spitzbubenschneider (Autodesk Fusion 360 design; units mm, degrees)
Autodesk Fusion 360 part; units mm, degrees
sketch "Sketch1" plane through (0, 0, 0) normal (0, 1, 0) x (1, 0, 0)
  circle A0 centre (0, 0) radius 27.5
  circle A1 centre (0, 0) radius 26.7
  circle A2 centre (14, 0) radius 4.05
  circle A3 centre (14, 0) radius 3.25
  line L0 (0, 0) -> (26.7, 0)
  line L1 (0, 0) -> (14, 0)
  circle A4 centre (14, 0) radius 6.45
  dimension "d1" = 55
  dimension "d2" = 0.8
  dimension "d3" = 0.8
  dimension "d4" = 14
  dimension "d5" = 6.5
  dimension "d43" = 2.4
  constraint coincident A0.centre A1.centre
  constraint concentric A2 A3
  constraint coincident A1 L0.end
  constraint horizontal L0
  constraint coincident A2.centre A3.centre
  constraint collinear L0 L1
  constraint concentric A3 A4
  measures "d1" diameter of A0
  measures "d2" distance of A0 A1
  measures "d3" distance of A2 A3
  measures "d4" distance of A0.centre A2.centre
  measures "d5" diameter of A3
  measures "d43" distance of A2 A4
extrude "Extrude1" add sketch "Sketch1" along normal blind 15 contours A0 | A2 A3 L0 L1 | A2 A3 L0 L1 makes body 1 at (27.3633, 10, 2.7381) makes body 2 at (18.0299, 5, 0.4032)
sketch "Sketch2" plane through (0, 0, 0) normal (0, 0, 1) x (1, 0, 0)
  line L0 (0, 0) -> (27.3, 0)
  line L1 (17.45, 0) -> (17.45, 3.4)
  line L2 (17.45, 3.4) -> (27.3, 0)
  line L3 (27.3, 0) -> (27.3, 3.4)
  line L4 (27.3, 3.4) -> (17.45, 3.4)
  line L5 (0, 0) -> (0, 3.4)
  line L6 (0, 3.4) -> (10.5, 3.4)
  line L7 (10.5, 3.4) -> (10.5, 0)
  dimension "d10" = 3.4
  dimension "d11" = 27.3
  dimension "d12" = 17.45
  dimension "d13" = 10.5
  constraint coincident L0.start L5.start
  constraint horizontal L0
  constraint coincident L0 L1.start
  constraint perpendicular L0 L1
  constraint perpendicular L0 L3
  constraint parallel L0 L4
  constraint perpendicular L0 L5
  constraint perpendicular L5 L6
  constraint coincident L0 L7.end
  constraint perpendicular L0 L7
  constraint collinear L4 L6
  measures "d10" distance of L1.start L1.end
  measures "d11" distance of L0.start L0.end
  measures "d12" distance of L0.start L1
  measures "d13" distance of L0.start L7
extrude "Extrude2" add sketch "Sketch2" along normal mid plane 2 separate body contours L0 L1 L2 | L2 L3 L4 makes body 3
pattern_circular "C-Pattern2" count 3 over 360 about axis through (0, 1.75, 0) along (0, 1, 0) of "Extrude1", "Extrude2" makes body 4 at (-11.3104, 5, -25.0664) makes body 5 at (-9.3642, 10, -15.4127) makes body 6 at (-9.5006, 1.1333, -18.4556) makes body 7 at (-16.053, 10, 22.3283) makes body 8 at (-8.6657, 10, 15.816) makes body 9 at (-11.2327, 1.1333, 17.4556)
sketch "Sketch4" plane through (0, 0, 0) normal (0, 0, 1) x (1, 0, 0)
  line L0 (0, 3.4) -> (-27.3, 3.4)
  line L1 (-27.3, 3.4) -> (-27.3, 0)
  line L2 (-27.3, 0) -> (0, 0)
  line L3 (0, 3.4) -> (0, 0)
  line L4 (-15, 0) -> (-15, 3.4)
  dimension "d20" = 3.4
  dimension "d22" = 27.3
  dimension "d42" = 15
  constraint vertical L1
  constraint coincident L2.end L3.end
  constraint perpendicular L1 L2
  constraint perpendicular L2 L3
  constraint coincident L2 L4.start
  constraint coincident L0 L4.end
  constraint perpendicular L0 L4
  measures "d20" distance of L0.end L1.end
  measures "d22" distance of L1 L3
  measures "d42" distance of L3 L4
extrude "Extrude3" add sketch "Sketch4" along normal mid plane 1.6 separate body contours L0 L1 L2 L4 makes body 10
pattern_circular "C-Pattern3" count 3 over 360 about axis through (0, 1.75, 0) along (0, 1, 0) of "Extrude3" makes body 11 at (10.2428, 2.2667, 16.1411) makes body 12 at (8.8572, 2.2667, -16.9411)
combine "Combine1" operation add target body 1 tool bodies 11 12 3 4 5 6 7 8 9 10 2
sketch "Sketch5" plane through (0, 0, 0) normal (0, 1, 0) x (1, 0, 0)
  circle A0 centre (0, 0) radius 27.375 construction
  circle A1 centre (0, 0) radius 27.375
  constraint coincident A0.centre A1.centre
sketch "Sketch6" plane through (0, 0, 0) normal (0, -1, 0) x (1, 0, 0)
  line L0 (8.1928, 12.5904) -> (14.0368, 22.7125)
  arc A0 (26.6813, 1) -> (14.0368, 22.7125) centre (0, 0) ccw
  line L1 (26.6813, 1) -> (17.9246, 1)
  circle A1 centre (14, 0) radius 3.25
  arc A2 (17.9246, 1) -> (17.9246, -1) centre (14, 0) ccw
  line L2 (17.9246, -1) -> (26.6813, -1)
  arc A3 (14.0368, -22.7125) -> (26.6813, -1) centre (0, 0) ccw
  line L3 (14.0368, -22.7125) -> (8.1928, -12.5904)
  arc A4 (-12.4746, -23.6067) -> (12.6512, -23.5125) centre (0, 0) ccw
  line L4 (-12.4746, -23.6067) -> (-8.0963, -16.0232)
  line L5 (6.8072, -13.3904) -> (12.6512, -23.5125)
  circle A5 centre (-7, -12.1244) radius 3.25
  circle A6 centre (0, 0) radius 27.5
  circle A7 centre (-7, 12.1244) radius 3.25
  line L6 (-8.0963, 16.0232) -> (-12.4746, 23.6067)
  arc A8 (12.6512, 23.5125) -> (-12.4746, 23.6067) centre (0, 0) ccw
  line L7 (12.6512, 23.5125) -> (6.8072, 13.3904)
  arc A9 (-9.8283, 15.0232) -> (-8.0963, 16.0232) centre (-7, 12.1244) ccw
  line L8 (-26.688, -0.8) -> (-15, -0.8)
  arc A10 (-8.0963, -16.0232) -> (-9.8283, -15.0232) centre (-7, -12.1244) ccw
  line L9 (-9.8283, -15.0232) -> (-14.2067, -22.6067)
  arc A11 (-26.688, -0.8) -> (-14.2067, -22.6067) centre (0, 0) ccw
  arc A12 (-14.2067, 22.6067) -> (-26.688, 0.8) centre (0, 0) ccw
  line L10 (-14.2067, 22.6067) -> (-9.8283, 15.0232)
  line L11 (-15, 0.8) -> (-26.688, 0.8)
  circle A13 centre (0, 0) radius 26.7
  line L12 (8.1928, -12.5904) -> (6.8072, -13.3904)
  line L13 (-15, -0.8) -> (-15, 0.8)
  line L14 (6.8072, 13.3904) -> (8.1928, 12.5904)
  constraint concentric A0 A13
  constraint coincident A3.start A13
sketch "Sketch8" plane through (-7, 0, 12.1244) normal (0, -1, 0) x (1, 0, 0)
  circle A0 centre (7, -12.1244) radius 15
  circle A1 centre (7, -12.1244) radius 13.4
  point P0 (7, -12.1244)
  dimension "d28" = 1.6
  dimension "d29" = 30
  constraint concentric A0 A1
  constraint coincident P0 A0.centre
  measures "d28" distance of A0 A1
  measures "d29" diameter of A0
extrude "Extrude4" add sketch "Sketch8" against normal blind 3.4 bodies 1
sketch "Sketch9" plane through (0, 0, 0) normal (0, -1, 0) x (1, 0, 0)
  circle A0 centre (0, 0) radius 29.5
  circle A1 centre (0, 0) radius 24.7
  circle A2 centre (0, 0) radius 26.7
  circle A3 centre (0, 0) radius 27.5
  dimension "d32" = 2
  dimension "d33" = 2
  constraint coincident A0.centre A1.centre
  measures "d32" distance of A1 A2
  measures "d33" distance of A0 A3
extrude "Extrude5" add sketch "Sketch9" against normal blind 3.4 bodies 1
fillet "Fillet1" [suppressed]
extrude "Extrude6" cut sketch "Sketch1" along normal blind 43 contours A3 L0 L1 | A3 L0 L1 bodies 1
pattern_circular "C-Pattern4" count 3 over 360 about axis through (0, 0, 0) along (0, 1, 0) of "Extrude6"
sketch "Sketch10" plane through (0, 0, 0) normal (0, 1, 0) x (1, 0, 0)
extrude "Extrude7" add sketch "Sketch1" along normal blind 3.4 contours A2 L0 L1 A4 | A2 L0 L1 A4 bodies 1
pattern_circular "C-Pattern5" count 3 over 360 about axis through (0, 1.75, 0) along (0, 1, 0) of "Extrude7"
equation "d3 = d2"
equation "d33 = d32"
named bodies: "Body3 (1)", "Body3 (2)"
